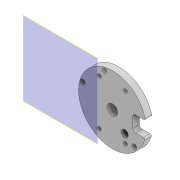
# Autodesk Inventor part: Anblerfish_middle2_v1
Saved by Autodesk Inventor 2022 (Build 260153000, 153)
## iProperties
Created: 2022-03-20
Part Number: Anblerfish_middle2_v1
Material: Generic
Document SubType Name: Modeling
Designer: Prakash Lab
Density: 1 g/cm^3
Appearance: Default
Author: Prakash Lab
Autodesk Inventor part; units mm, degrees
ref_plane "YZ Plane" through (0, 0, 0) normal (1, 0, 0) x (0, 1, 0)
ref_plane "XZ Plane" through (0, 0, 0) normal (0, 1, 0) x (-1, 0, 0)
ref_plane "XY Plane" through (0, 0, 0) normal (0, 0, 1) x (1, 0, 0)
ref_plane "Work Plane1" through (-54.651493, -58.936858, 28.800864) normal (0, 0, -1) x (-1, 0, 0)
sketch "Sketch1" plane through (-50.651398, -58.936858, 28.800864) normal (0, 0, 1) x (1, 0, 0)
  circle A0 centre (-11.999881, -12.497897) radius 25.997895
  circle A1 centre (-2.000047, 4.999944) radius 1.399928
  circle A2 centre (-22.000015, 4.999967) radius 1.399965
  circle A3 centre (-12, -12.50005) radius 3.85005
  line L0 (-5.000001, -5) -> (-5.000001, 0)
  line L1 (0, 0) -> (0, -5)
  circle A4 centre (-21.999984, -30) radius 1.399983
  circle A5 centre (-2.000029, -29.999956) radius 1.400053
  line L2 (-5.000001, 0) -> (0, 0)
  line L3 (0, 0) -> (0, -5)
  line L4 (0, -5) -> (-5.000001, -5)
  line L5 (-5.000001, -5) -> (-5.000001, 0)
  circle A6 centre (-12, -12.50005) radius 4
  point P0 (50.651398, 58.936858)
  dimension "d2" = 8
  constraints: 8 end point, 2 parallel, 1 centre point, 1 coincident, 1 horizontal, 1 perpendicular
  measures "d2" diameter of A6
sketch "Sketch1 outline for Extrusion1" plane through (-50.651398, -58.936858, 28.800864) normal (0, 0, 1) x (1, 0, 0)
  circle A0 centre (-11.999881, -12.497897) radius 25.997895
  circle A1 centre (-21.999984, -30) radius 1.399983
  circle A2 centre (-2.000029, -29.999956) radius 1.400053
  circle A3 centre (-22.000015, 4.999967) radius 1.399965
  circle A4 centre (-2.000047, 4.999944) radius 1.399928
extrude "Extrusion1" add sketch "Sketch1 outline for Extrusion1" against normal blind 5
sketch "Sketch2" plane through (-62.651279, -71.434756, 28.800864) normal (0, 0, 1) x (1, 0, 0)
  circle A0 centre (-0.00012, -0.002152) radius 3.85005
  circle A1 centre (-0.00012, -0.002152) radius 3.95
  point P0 (62.651279, 71.434756)
  dimension "d3" = 7.9
  constraints: 1 centre point, 1 coincident
  measures "d3" diameter of A1
sketch "Sketch2 outline for Extrusion2" plane through (-62.651279, -71.434756, 28.800864) normal (0, 0, 1) x (1, 0, 0)
  circle A0 centre (-0.00012, -0.002152) radius 3.95
extrude "Extrusion2" cut sketch "Sketch2 outline for Extrusion2" against normal blind 25.4 draft -2
ref_plane "Arbeitsebene4" through (-62.651279, -71.434756, 23.790864) normal (0, 0, -1) x (-1, 0, 0)
sketch "Sketch7" plane through (-62.651279, -71.434756, 23.790864) normal (0, 0, -1) x (-1, 0, 0)
  circle A0 centre (-16.829084, -16.048143) radius 2.45
  circle A1 centre (-9.499801, -11.002158) radius 2.660104
  circle A2 centre (-16.829084, -16.048143) radius 1.4
  point P0 (-62.651279, 71.434756)
  dimension "d30" = 2.8
  constraints: 1 centre point, 1 coincident
  measures "d30" diameter of A2
sketch "Sketch7 outline for Extrusion5" plane through (-62.651279, -71.434756, 23.790864) normal (0, 0, -1) x (-1, 0, 0)
  circle A0 centre (-16.829084, -16.048143) radius 1.4
  circle A1 centre (-9.499801, -11.002158) radius 2.660104
extrude "Extrusion5" cut sketch "Sketch7 outline for Extrusion5" against normal through all
ref_plane "Arbeitsebene3" through (-62.651279, -71.434756, 23.790864) normal (0, 0, -1) x (-1, 0, 0)
sketch "Sketch8" plane through (-62.651279, -71.434756, 23.790864) normal (0, 0, -1) x (-1, 0, 0)
  line L0 (19.658141, 5.145881) -> (6.483141, 5.145881)
  circle A0 centre (0, 0) radius 23.822
  circle A1 centre (22.711924, 7.187224) radius 1.75
  circle A2 centre (6.128376, 23.020224) radius 1.75
  circle A3 centre (-16.829084, -16.048143) radius 1.4
  circle A4 centre (-16.829084, -16.048143) radius 1.75
  point P0 (-62.651279, 71.434756)
  dimension "d33" = 3.5
  dimension "d34" = 3.5
  dimension "d60" = 47.644
  dimension "d61" = 2.04134
  dimension "d62" = 17.87434
  dimension "d63" = 3.5
  constraints: 4 centre point, 2 end point, 2 point on circle, 1 coincident, 1 horizontal, 2 other
  measures "d33" diameter of A1
  measures "d34" diameter of A2
  measures "d60" diameter of A0
  measures "d61" distance from line of A1.centre L0
  measures "d62" distance from line of A2.centre L0
  measures "d63" diameter of A4
sketch "Sketch8 outline for Extrusion6" plane through (-62.651279, -71.434756, 23.790864) normal (0, 0, -1) x (-1, 0, 0)
  circle A0 centre (22.711924, 7.187224) radius 1.75
  circle A1 centre (6.128376, 23.020224) radius 1.75
  circle A2 centre (-16.829084, -16.048143) radius 1.75
extrude "Extrusion6" cut sketch "Sketch8 outline for Extrusion6" against normal through all
ref_plane "Arbeitsebene2" through (-62.651279, -71.434756, 23.790864) normal (0, 0, -1) x (-1, 0, 0)
sketch "Sketch9" plane through (-62.651279, -71.434756, 23.790864) normal (0, 0, -1) x (-1, 0, 0)
  line L0 (15.077087, 22.687708) -> (22.406392, 9.030062)
  arc A0 (-25.107353, 6.751423) -> (-24.141678, 5.49167) centre (-24.141678, 6.49167) ccw
  arc A1 (-23.850222, -6.495985) -> (-24.804238, -7.795738) centre (-23.850222, -7.495985) ccw
  line L1 (-21.499801, -6.495985) -> (-23.850222, -6.495985)
  line L2 (-24.141678, 5.49167) -> (-21.499801, 5.49167)
  circle A2 centre (0, 0) radius 25.997895
  line L3 (-15.700236, 3.49167) -> (-15.700236, -4.495985)
  line L4 (-17.700236, -6.495985) -> (-21.499801, -6.495985)
  line L5 (-21.499801, 5.49167) -> (-17.700236, 5.49167)
  arc A3 (-15.700236, 3.49167) -> (-17.700236, 5.49167) centre (-17.700236, 3.49167) ccw
  arc A4 (-17.700236, -6.495985) -> (-15.700236, -4.495985) centre (-17.700236, -4.495985) ccw
  point P0 (-62.651279, 71.434756)
  point P1 (-25.119784, 6.699776)
  point P2 (-24.823544, -7.725425)
  dimension "d37" = 2
  constraints: 12 end point, 8 point on circle, 4 centre point, 4 tangent, 2 horizontal, 1 equal radius, 1 parallel, 1 perpendicular, 1 vertical, 13 other
  measures "d37" radius of A3
sketch "Sketch9 outline for Extrusion7" plane through (-62.651279, -71.434756, 23.790864) normal (0, 0, -1) x (-1, 0, 0)
  line L0 (-23.850222, -6.495985) -> (-21.499801, -6.495985)
  arc A0 (-24.823544, -7.725425) -> (-23.850222, -6.495985) centre (-23.850222, -7.495985) cw
  arc A1 (-25.119784, 6.699776) -> (-24.823544, -7.725425) centre (0, 0) ccw
  arc A2 (-24.141678, 5.49167) -> (-25.119784, 6.699776) centre (-24.141678, 6.49167) cw
  line L1 (-21.499801, 5.49167) -> (-24.141678, 5.49167)
  line L2 (-17.700236, 5.49167) -> (-21.499801, 5.49167)
  arc A3 (-15.700236, 3.49167) -> (-17.700236, 5.49167) centre (-17.700236, 3.49167) ccw
  line L3 (-15.700236, -4.495985) -> (-15.700236, 3.49167)
  arc A4 (-17.700236, -6.495985) -> (-15.700236, -4.495985) centre (-17.700236, -4.495985) ccw
  line L4 (-21.499801, -6.495985) -> (-17.700236, -6.495985)
extrude "Extrusion7" cut sketch "Sketch9 outline for Extrusion7" against normal through all
sketch "Skizze12" plane through (-50.651398, -58.936858, 23.800864) normal (0, 0, -1) x (-1, 0, 0)
  line L0 (27.279321, -9.665289) -> (37.905021, -9.665289) construction
  line L1 (37.905021, -9.665289) -> (37.905021, -14.123191) construction
  line L2 (37.905021, -14.123191) -> (27.279321, -14.123191) construction
  line L3 (27.279321, -14.123191) -> (27.279321, -9.665289) construction
  spline S0 degree 2 poles (29.597716, -15.982794) (28.935318, -15.982794) (28.005982, -15.705971) (27.59569, -15.50824) knots 0 0 0 1 2 2 2
  line L4 (27.59569, -15.50824) -> (27.59569, -14.489925)
  line L5 (27.59569, -14.489925) -> (27.65501, -14.489925)
  spline S1 degree 2 poles (27.65501, -14.489925) (28.055415, -14.865614) (29.068786, -15.280849) (29.538397, -15.280849) knots 0 0 0 1 2 2 2
  spline S2 degree 2 poles (29.538397, -15.280849) (30.210682, -15.280849) (30.897797, -14.722259) (30.897797, -14.262535) knots 0 0 0 1 2 2 2
  spline S3 degree 2 poles (30.897797, -14.262535) (30.897797, -13.896732) (30.536938, -13.441951) (30.14642, -13.328256) knots 0 0 0 1 2 2 2
  spline S4 degree 2 poles (30.14642, -13.328256) (29.864653, -13.249163) (29.395042, -13.140411) (29.04407, -13.051432) knots 0 0 0 1 2 2 2
  spline S5 degree 2 poles (29.04407, -13.051432) (28.7277, -12.967397) (28.228429, -12.71529) (28.035642, -12.512616) knots 0 0 0 1 2 2 2
  spline S6 degree 2 poles (28.035642, -12.512616) (27.847797, -12.309941) (27.64018, -11.766181) (27.64018, -11.410265) knots 0 0 0 1 2 2 2
  spline S7 degree 2 poles (27.64018, -11.410265) (27.64018, -10.668774) (28.796906, -9.66529) (29.691639, -9.66529) knots 0 0 0 1 2 2 2
  spline S8 degree 2 poles (29.691639, -9.66529) (30.205739, -9.66529) (31.115301, -9.867964) (31.50582, -10.060752) knots 0 0 0 1 2 2 2
  line L6 (31.50582, -10.060752) -> (31.50582, -11.029633)
  line L7 (31.50582, -11.029633) -> (31.446501, -11.029633)
  spline S9 degree 2 poles (31.446501, -11.029633) (31.154848, -10.762697) (30.245285, -10.367235) (29.746015, -10.367235) knots 0 0 0 1 2 2 2
  spline S10 degree 2 poles (29.746015, -10.367235) (29.182481, -10.367235) (28.48548, -10.896165) (28.48548, -11.32623) knots 0 0 0 1 2 2 2
  spline S11 degree 2 poles (28.48548, -11.32623) (28.48548, -11.711805) (28.895771, -12.17153) (29.281347, -12.275338) knots 0 0 0 1 2 2 2
  spline S12 degree 2 poles (29.281347, -12.275338) (29.538397, -12.344544) (30.284831, -12.522502) (30.531995, -12.596651) knots 0 0 0 1 2 2 2
  spline S13 degree 2 poles (30.531995, -12.596651) (31.159791, -12.789439) (31.743097, -13.565533) (31.743097, -14.134009) knots 0 0 0 1 2 2 2
  spline S14 degree 2 poles (31.743097, -14.134009) (31.743097, -14.494868) (31.451444, -15.186927) (31.189451, -15.429147) knots 0 0 0 1 2 2 2
  spline S15 degree 2 poles (31.189451, -15.429147) (30.897797, -15.696084) (30.156306, -15.982794) (29.597716, -15.982794) knots 0 0 0 1 2 2 2
  spline S16 degree 2 poles (37.37843, -12.828985) (37.37843, -13.664398) (36.701201, -15.008969) (36.132725, -15.384658) knots 0 0 0 1 2 2 2
  spline S17 degree 2 poles (36.132725, -15.384658) (35.668057, -15.676311) (34.714005, -15.874042) (33.972514, -15.874042) knots 0 0 0 1 2 2 2
  line L8 (33.972514, -15.874042) -> (32.568624, -15.874042)
  line L9 (32.568624, -15.874042) -> (32.568624, -9.774042)
  line L10 (32.568624, -9.774042) -> (33.957684, -9.774042)
  spline S18 degree 2 poles (33.957684, -9.774042) (34.817814, -9.774042) (35.796582, -10.031092) (36.142611, -10.258483) knots 0 0 0 1 2 2 2
  spline S19 degree 2 poles (36.142611, -10.258483) (36.730861, -10.649001) (37.37843, -11.939196) (37.37843, -12.828985) knots 0 0 0 1 2 2 2
  spline S20 degree 2 poles (36.53313, -12.819099) (36.53313, -12.117154) (36.068462, -11.123556) (35.608738, -10.841789) knots 0 0 0 1 2 2 2
  spline S21 degree 2 poles (35.608738, -10.841789) (35.282481, -10.649001) (34.545934, -10.475987) (33.99723, -10.475987) knots 0 0 0 1 2 2 2
  line L11 (33.99723, -10.475987) -> (33.379321, -10.475987)
  line L12 (33.379321, -10.475987) -> (33.379321, -15.172097)
  line L13 (33.379321, -15.172097) -> (33.99723, -15.172097)
  spline S22 degree 2 poles (33.99723, -15.172097) (34.536047, -15.172097) (35.351687, -14.999082) (35.682887, -14.766748) knots 0 0 0 1 2 2 2
  spline S23 degree 2 poles (35.682887, -14.766748) (36.108008, -14.480039) (36.53313, -13.53093) (36.53313, -12.819099) knots 0 0 0 1 2 2 2
  point P0 (-50.651398, 58.936858)
  constraints: 2 other
sketch "Skizze12 outline for Extrusion10" plane through (-50.651398, -58.936858, 23.800864) normal (0, 0, -1) x (-1, 0, 0)
  spline S0 degree 2 poles (29.597716, -15.982794) (28.935318, -15.982794) (28.005982, -15.705971) (27.59569, -15.50824) knots 0 0 0 0.5 1 1 1
  line L0 (27.59569, -15.50824) -> (27.59569, -14.489925)
  line L1 (27.59569, -14.489925) -> (27.65501, -14.489925)
  spline S1 degree 2 poles (27.65501, -14.489925) (28.055415, -14.865614) (29.068786, -15.280849) (29.538397, -15.280849) knots 0 0 0 0.5 1 1 1
  spline S2 degree 2 poles (29.538397, -15.280849) (30.210682, -15.280849) (30.897797, -14.722259) (30.897797, -14.262535) knots 0 0 0 0.5 1 1 1
  spline S3 degree 2 poles (30.897797, -14.262535) (30.897797, -13.896732) (30.536938, -13.441951) (30.14642, -13.328256) knots 0 0 0 0.5 1 1 1
  spline S4 degree 2 poles (30.14642, -13.328256) (29.864653, -13.249163) (29.395042, -13.140411) (29.04407, -13.051432) knots 0 0 0 0.5 1 1 1
  spline S5 degree 2 poles (29.04407, -13.051432) (28.7277, -12.967397) (28.228429, -12.71529) (28.035642, -12.512616) knots 0 0 0 0.5 1 1 1
  spline S6 degree 2 poles (28.035642, -12.512616) (27.847797, -12.309941) (27.64018, -11.766181) (27.64018, -11.410265) knots 0 0 0 0.5 1 1 1
  spline S7 degree 2 poles (27.64018, -11.410265) (27.64018, -10.668774) (28.796906, -9.66529) (29.691639, -9.66529) knots 0 0 0 0.5 1 1 1
  spline S8 degree 2 poles (29.691639, -9.66529) (30.205739, -9.66529) (31.115301, -9.867964) (31.50582, -10.060752) knots 0 0 0 0.5 1 1 1
  line L2 (31.50582, -10.060752) -> (31.50582, -11.029633)
  line L3 (31.50582, -11.029633) -> (31.446501, -11.029633)
  spline S9 degree 2 poles (31.446501, -11.029633) (31.154848, -10.762697) (30.245285, -10.367235) (29.746015, -10.367235) knots 0 0 0 0.5 1 1 1
  spline S10 degree 2 poles (29.746015, -10.367235) (29.182481, -10.367235) (28.48548, -10.896165) (28.48548, -11.32623) knots 0 0 0 0.5 1 1 1
  spline S11 degree 2 poles (28.48548, -11.32623) (28.48548, -11.711805) (28.895771, -12.17153) (29.281347, -12.275338) knots 0 0 0 0.5 1 1 1
  spline S12 degree 2 poles (29.281347, -12.275338) (29.538397, -12.344544) (30.284831, -12.522502) (30.531995, -12.596651) knots 0 0 0 0.5 1 1 1
  spline S13 degree 2 poles (30.531995, -12.596651) (31.159791, -12.789439) (31.743097, -13.565533) (31.743097, -14.134009) knots 0 0 0 0.5 1 1 1
  spline S14 degree 2 poles (31.743097, -14.134009) (31.743097, -14.494868) (31.451444, -15.186927) (31.189451, -15.429147) knots 0 0 0 0.5 1 1 1
  spline S15 degree 2 poles (31.189451, -15.429147) (30.897797, -15.696084) (30.156306, -15.982794) (29.597716, -15.982794) knots 0 0 0 0.5 1 1 1
  spline S16 degree 2 poles (37.37843, -12.828985) (37.37843, -13.664398) (36.701201, -15.008969) (36.132725, -15.384658) knots 0 0 0 0.5 1 1 1
  spline S17 degree 2 poles (36.142611, -10.258483) (36.730861, -10.649001) (37.37843, -11.939196) (37.37843, -12.828985) knots 0 0 0 0.5 1 1 1
  spline S18 degree 2 poles (36.132725, -15.384658) (35.668057, -15.676311) (34.714005, -15.874042) (33.972514, -15.874042) knots 0 0 0 0.5 1 1 1
  spline S19 degree 2 poles (33.957684, -9.774042) (34.817814, -9.774042) (35.796582, -10.031092) (36.142611, -10.258483) knots 0 0 0 0.5 1 1 1
  line L4 (33.972514, -15.874042) -> (32.568624, -15.874042)
  line L5 (32.568624, -9.774042) -> (33.957684, -9.774042)
  line L6 (32.568624, -15.874042) -> (32.568624, -9.774042)
  spline S20 degree 2 poles (35.682887, -14.766748) (36.108008, -14.480039) (36.53313, -13.53093) (36.53313, -12.819099) knots 0 0 0 0.5 1 1 1
  spline S21 degree 2 poles (36.53313, -12.819099) (36.53313, -12.117154) (36.068462, -11.123556) (35.608738, -10.841789) knots 0 0 0 0.5 1 1 1
  spline S22 degree 2 poles (35.608738, -10.841789) (35.282481, -10.649001) (34.545934, -10.475987) (33.99723, -10.475987) knots 0 0 0 0.5 1 1 1
  line L7 (33.99723, -10.475987) -> (33.379321, -10.475987)
  line L8 (33.379321, -10.475987) -> (33.379321, -15.172097)
  line L9 (33.379321, -15.172097) -> (33.99723, -15.172097)
  spline S23 degree 2 poles (33.99723, -15.172097) (34.536047, -15.172097) (35.351687, -14.999082) (35.682887, -14.766748) knots 0 0 0 0.5 1 1 1
extrude "Extrusion10" cut sketch "Skizze12 outline for Extrusion10" against normal blind 1
sketch "Skizze13" plane through (-50.651398, -58.936858, 23.800864) normal (0, 0, -1) x (-1, 0, 0)
  circle A0 centre (12, -12.50005) radius 3.775396 construction
  circle A1 centre (12, -12.50005) radius 3.35
  circle A2 centre (12, -12.50005) radius 5
  point P0 (-50.651398, 58.936858)
  dimension "d53" = 6.7
  dimension "d54" = 10
  constraints: 2 centre point, 2 coincident
  measures "d53" diameter of A1
  measures "d54" diameter of A2
sketch "Skizze13 outline for Extrusion11" plane through (-50.651398, -58.936858, 23.800864) normal (0, 0, -1) x (-1, 0, 0)
  circle A0 centre (12, -12.50005) radius 5
  circle A1 centre (12, -12.50005) radius 3.35
extrude "Extrusion11" add sketch "Skizze13 outline for Extrusion11" along normal blind 4
chamfer "Fase3" distance 1.5 angle 45 2 edges at (-57.6514, -71.4369, 19.8009) (-57.6514, -71.4369, 23.8009)
body "Solid1"
